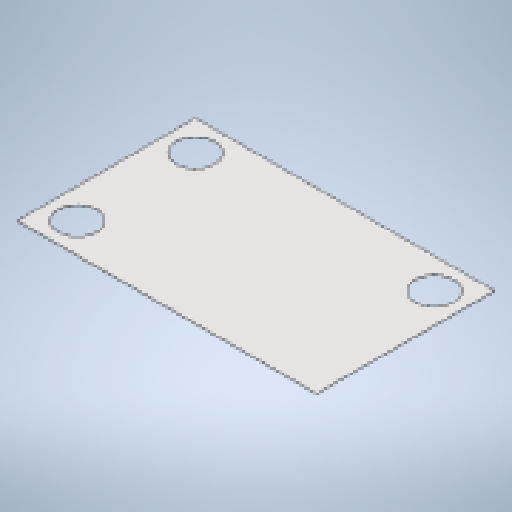
# Autodesk Inventor part: GBK-RK-0021 bottom
Saved by Autodesk Inventor 2026.2 (Build 302298000, 298)
## iProperties
Created: 2026-09-14
Part Number: GBK-RK-0021 bottom
Material: Generic
Document SubType Name: Sheet Metal
Designer: admin
Density: 1 g/cm^3
Sheet Metal Rule: Default
Appearance: Default
Author: admin
Autodesk Inventor part; units mm, degrees
ref_plane "YZ Plane" through (0, 0, 0) normal (1, 0, 0) x (0, 1, 0)
ref_plane "XZ Plane" through (0, 0, 0) normal (0, 1, 0) x (-1, 0, 0)
ref_plane "XY Plane" through (0, 0, 0) normal (0, 0, 1) x (1, 0, 0)
sketch "Sketch1" plane through (0, 0, 0) normal (0, 1, 0) x (-1, 0, 0)
  line L0 (1244, -740) -> (-1244, -740)
  line L1 (-1244, -740) -> (-1244, 740)
  line L2 (-1244, 740) -> (1244, 740)
  line L3 (1244, 740) -> (1244, -740)
  line L4 (1244, -740) -> (-1244, 740) construction
  line L5 (-1244, -740) -> (1244, 740) construction
  point P0 (0, 0)
  dimension "d0" = 2488
  dimension "d1" = 1480
  measures "d0" distance of L1.end L2.end
  measures "d1" distance of L0.end L1.end
extrude "Plate1" add sketch "Sketch1" along normal blind 4
sketch "Sketch2" plane through (0, 4, 0) normal (0, 1, 0) x (1, 0, 0)
  line L0 (-1244, -740) -> (-1244, 740) construction
  line L1 (1244, -740) -> (-1244, -740) construction
  line L2 (1244, 740) -> (1244, -740) construction
  line L3 (-1244, 740) -> (1244, 740) construction
  circle A0 centre (-994, 490) radius 162.5
  point P0 (0, 0)
  dimension "d6" = 325
  dimension "d7" = 250
  dimension "d8" = 250
  constraints: 1 centre point
  measures "d6" diameter of A0
  measures "d7" distance from line of A0.centre L0
  measures "d8" distance from line of A0.centre L3
extrude "Cut1" cut sketch "Sketch2" against normal blind 4
mirror "Mirror1" about plane through (0, 0, 0) normal (1, 0, 0) of "Cut1"
mirror "Mirror2" about plane through (0, 0, 0) normal (0, 0, 1) of "Cut1"
fillet "Corner Round1" radius 20 4 edges at (-1244, 2, 740) (-1244, 2, -740) (1244, 2, -740) (1244, 2, 740)
equation "\"d9\" = Thickness"
equation "\"d2\" = Thickness"
equation "\"BendRadius\" = Thickness"
equation "\"BendReliefWidth\" = Thickness"
equation "\"BendReliefDepth\" = 0.5 * Thickness"
equation "\"CornerReliefSize\" = 4 * Thickness"
equation "\"MinimumRemnant\" = 2 * Thickness"
equation "\"TransitionRadius\" = BendRadius"
equation "\"JacobiRadiusSize\" = BendRadius"
equation "\"GapSize\" = Thickness"
equation "\"Thickness\" = 4"
body "Solid1"
